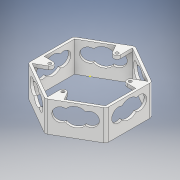
# Autodesk Inventor part: radar
Saved by Autodesk Inventor 2018 (Build 220112000, 112)
## iProperties
Created: 2017-05-12
Part Number: radar
Material: Default New Material(1)
Document SubType Name: Modeling
Designer: Vidal Villegas
Density: 1.13872 g/cm^3
Appearance: PLA
Mass: 28.1682 g
Surface Area: 205.405 cm^2
Volume: 24.7367 cm^3
Author: Vidal Villegas
Autodesk Inventor part; units mm, degrees
ref_plane "YZ Plane" through (0, 0, 0) normal (1, 0, 0) x (0, 1, 0)
ref_plane "XZ Plane" through (0, 0, 0) normal (0, 1, 0) x (-1, 0, 0)
ref_plane "XY Plane" through (0, 0, 0) normal (0, 0, 1) x (1, 0, 0)
sketch "Sketch1" plane through (0, 0, 0) normal (0, 0, 1) x (1, 0, 0)
  line L0 (-47.5136, -27.432) -> (-47.5136, 27.432)
  line L1 (-47.5136, 27.432) -> (0, 54.864)
  line L2 (0, 54.864) -> (47.5136, 27.432)
  line L3 (47.5136, 27.432) -> (47.5136, -27.432)
  line L4 (47.5136, -27.432) -> (0, -54.864)
  line L5 (0, -54.864) -> (-47.5136, -27.432)
  line L6 (0, 51.3999) -> (44.5136, 25.6999)
  line L7 (44.5136, 25.6999) -> (44.5136, -25.6999)
  line L8 (44.5136, -25.6999) -> (0, -51.3999)
  line L9 (0, -51.3999) -> (-44.5136, -25.6999)
  line L10 (-44.5136, -25.6999) -> (-44.5136, 25.6999)
  line L11 (-44.5136, 25.6999) -> (0, 51.3999)
  point P0 (0, 0)
  point P1 (0, 0)
  point P2 (0, 0)
  dimension "d0" = 54.864
  dimension "d1" = 3
  constraints: 24 end point, 2 coincident, 2 vertical alignment, 26 other
  measures "d0" distance of L0.start L0.end
  measures "d1" distance between parallel lines of L1 L11
extrude "Extrusion1" add sketch "Sketch1" along normal blind 37
sketch "Sketch2" plane through (0, 0, 37) normal (0, 0, 1) x (1, 0, 0)
  line L0 (0, 51.3999) -> (44.5136, 25.6999) projected
  line L1 (44.5136, 25.6999) -> (44.5136, -25.6999) projected
  line L2 (44.5136, -25.6999) -> (0, -51.3999) projected
  line L3 (0, -51.3999) -> (-44.5136, -25.6999) projected
  line L4 (-44.5136, -25.6999) -> (-44.5136, 25.6999) projected
  line L5 (-44.5136, 25.6999) -> (0, 51.3999) projected
  line L6 (-29.2636, 16.8954) -> (0, 33.7907)
  line L7 (0, 33.7907) -> (29.2636, 16.8954)
  line L8 (29.2636, 16.8954) -> (29.2636, -16.8954)
  line L9 (29.2636, -16.8954) -> (0, -33.7907)
  line L10 (0, -33.7907) -> (-29.2636, -16.8954)
  line L11 (-29.2636, -16.8954) -> (-29.2636, 16.8954)
  point P0 (0, 0)
  point P1 (0, 0)
  dimension "d4" = 15.25
  constraints: 12 end point, 1 coincident, 1 vertical alignment, 13 other
  measures "d4" distance between parallel lines of L8 L1
extrude "Extrusion2" add sketch "Sketch2" against normal blind 4
sketch "Sketch5" plane through (0, 0, 33) normal (0, 0, -1) x (-1, 0, 0)
  point P0 (0, 0)
sketch "Sketch6" plane through (0, 54.864, 37) normal (0.5, 0.8660254, 0) x (0.8660254, -0.5, 0)
  circle A0 centre (14.682, 14.5) radius 8.44
  circle A1 centre (40.182, 14.5) radius 8.44
  line L0 (0, 37) -> (54.864, 37) projected
  line L1 (0, 37) -> (0, 0) projected
  line L2 (54.864, 0) -> (0, 0) projected
  line L3 (54.864, 37) -> (54.864, 0) projected
  arc A2 (15.7427, 14.5) -> (39.1213, 14.5) centre (27.432, 15) ccw
  arc A3 (39.1213, 14.5) -> (15.7427, 14.5) centre (27.432, 14) ccw
  line L4 (27.432, 37) -> (27.432, 28.8885) construction
  point P0 (27.432, 37)
  dimension "d49" = 25.5
  dimension "d51" = 8.44
  dimension "d53" = 11.7
  dimension "d54" = 15
  dimension "d55" = 23
  dimension "d58" = 14.5
  constraints: 4 centre point, 4 point on circle, 2 end point, 2 equal radius, 2 vertical alignment, 1 horizontal alignment, 1 midpoint, 1 symmetric about line, 1 vertical
  measures "d49" distance of A0.centre A1.centre
  measures "d51" radius of A1
  measures "d53" radius of A2
  measures "d54" distance from line of A2.centre L2
  measures "d55" distance from line of L0 A3.centre
  measures "d58" distance from line of A0.centre L2
extrude "Extrusion3" cut sketch "Sketch6" against normal through all contours A0 A2 A3 | A0 A3 A1 A2 | A3 A2 A0 | A3 A2 A1 | A1 A2 A3
sketch "Sketch7" plane through (47.5136, -27.432, 0) normal (1, 0, 0) x (0, 0, -1)
  line L0 (0, 54.864) -> (0, 0) projected
  line L1 (0, 54.864) -> (-37, 54.864) projected
  line L2 (-37, 0) -> (-37, 54.864) projected
  line L3 (0, 0) -> (-37, 0) projected
  circle A0 centre (-22.5, 40.932) radius 8.5
  circle A1 centre (-22.5, 13.932) radius 8.5
  arc A2 (-17.5, 17.3946) -> (-17.5, 37.4694) centre (-13, 27.432) ccw
  arc A3 (-17.5, 37.4694) -> (-17.5, 17.3946) centre (-22, 27.432) ccw
  line L4 (0, 53.1319) -> (0, 1.7321) construction
  line L5 (0, 27.432) -> (3.1756, 27.432) construction
  point P0 (48.3121, 34.9149)
  point P1 (0, 27.432)
  dimension "d66" = 8.5
  dimension "d67" = 27
  dimension "d68" = 14.5
  dimension "d70" = 22
  dimension "d71" = 15
  dimension "d72" = 13
  constraints: 4 centre point, 4 point on circle, 2 end point, 2 equal radius, 2 horizontal alignment, 2 midpoint, 1 horizontal, 1 symmetric about line, 1 vertical alignment
  measures "d66" radius of A1
  measures "d67" distance of A0.centre A1.centre
  measures "d68" distance from line of L2 A0.centre
  measures "d70" diameter of A2
  measures "d71" distance from line of L2 A3.centre
  measures "d72" distance from line of A2.centre L0
extrude "Extrusion4" [suppressed]
sketch "Sketch8" plane through (47.5136, -27.432, 0) normal (0.5, -0.8660254, 0) x (0.8660254, 0.5, 0)
  line L0 (-54.864, 0) -> (0, 0) projected
  line L1 (-54.864, 0) -> (-54.864, 37) projected
  line L2 (0, 37) -> (-54.864, 37) projected
  line L3 (0, 0) -> (0, 37) projected
  line L4 (-54.864, 0) -> (0, 0) projected
  line L5 (-54.864, 0) -> (-54.864, 37) projected
  line L6 (0, 37) -> (-54.864, 37) projected
  line L7 (0, 0) -> (0, 37) projected
  circle A0 centre (13.932, 22.5) radius 8.5
  circle A1 centre (40.932, 22.5) radius 8.5
  line L8 (0, 37) -> (54.864, 37)
  line L9 (0, 37) -> (0, 0)
  line L10 (54.864, 0) -> (0, 0)
  line L11 (54.864, 37) -> (54.864, 0)
  arc A2 (17.3946, 17.5) -> (37.4694, 17.5) centre (27.432, 13) ccw
  arc A3 (37.4694, 17.5) -> (17.3946, 17.5) centre (27.432, 22) ccw
  line L12 (27.432, 37) -> (27.432, 28.8885) construction
  circle A4 centre (-13.932, 22.5) radius 8.5
  circle A5 centre (-40.932, 22.5) radius 8.5
  line L13 (0, 37) -> (-54.864, 37)
  line L14 (-54.864, 0) -> (0, 0)
  line L15 (-54.864, 37) -> (-54.864, 0)
  arc A6 (-37.4694, 17.5) -> (-17.3946, 17.5) centre (-27.432, 13) ccw
  arc A7 (-17.3946, 17.5) -> (-37.4694, 17.5) centre (-27.432, 22) ccw
  line L16 (-27.432, 37) -> (-27.432, 28.8885) construction
  line L17 (27.432, 0) -> (0, 0) projected
  line L18 (27.432, 0) -> (27.432, 37) projected
  line L19 (0, 37) -> (27.432, 37) projected
  line L20 (0, 0) -> (0, 37) projected
  line L21 (0, 0) -> (-54.864, 0) projected
  line L22 (-54.864, 37) -> (0, 37) projected
  line L23 (0, 0) -> (0, 37) projected
  point P0 (-27.432, 0)
  point P1 (27.432, 27)
  point P2 (-27.432, 27)
  dimension "d75" = 27
  dimension "d76" = 8.5
  dimension "d77" = 11
  dimension "d78" = 13
  dimension "d79" = 15
  dimension "d81" = 14.5
  dimension "d82" = 54.864
  dimension "d83" = 54.864
  constraints: 18 end point, 10 symmetric about line, 8 centre point, 8 point on circle, 2 collinear, 2 equal radius, 2 vertical, 2 vertical alignment, 1 horizontal, 1 horizontal alignment, 1 midpoint, 5 other
  measures "d75" distance of A0.centre A1.centre
  measures "d76" radius of A1
  measures "d77" radius of A2
  measures "d78" distance from line of A2.centre L10
  measures "d79" distance from line of L8 A3.centre
  measures "d81" distance from line of A0.centre L8
  measures "d82" distance between parallel lines of L9 L1
  measures "d83" distance between parallel lines of L3 L11
extrude "Extrusion5" [suppressed]
sketch "Sketch9" plane through (0, 0, 33) normal (0, 0, -1) x (-1, 0, 0)
  line L0 (0, 54.805) -> (-47.4625, 27.4025)
  line L1 (-47.4625, 27.4025) -> (-47.4625, -27.4025)
  line L2 (-47.4625, -27.4025) -> (0, -54.805)
  line L3 (-47.4625, 27.4025) -> (0, 54.805)
  line L4 (0, 54.805) -> (47.4625, 27.4025)
  line L5 (47.4625, 27.4025) -> (47.4625, -27.4025)
  line L6 (47.4625, -27.4025) -> (0, -54.805)
  line L7 (0, -54.805) -> (-47.4625, -27.4025)
  line L8 (-47.4625, -27.4025) -> (-47.4625, 27.4025)
  circle A0 centre (-29.8779, -21.75) radius 1.55
  circle A1 centre (-33.775, -15) radius 1.55
  circle A2 centre (-33.775, 15) radius 1.55
  circle A3 centre (-3.8971, -36.75) radius 1.55
  circle A4 centre (3.8971, -36.75) radius 1.55
  circle A5 centre (29.8779, -21.75) radius 1.55
  circle A6 centre (33.775, -15) radius 1.55
  circle A7 centre (33.775, 15) radius 1.55
  circle A8 centre (29.8779, 21.75) radius 1.55
  circle A9 centre (3.8971, 36.75) radius 1.55
  circle A10 centre (-3.8971, 36.75) radius 1.55
  line L9 (-33.775, 19.5) -> (0, 39) construction
  line L10 (0, 39) -> (33.775, 19.5) construction
  line L11 (33.775, 19.5) -> (33.775, -19.5) construction
  line L12 (33.775, -19.5) -> (0, -39) construction
  line L13 (0, -39) -> (-33.775, -19.5) construction
  line L14 (-33.775, -19.5) -> (-33.775, 19.5) construction
  circle A11 centre (-29.8779, 21.75) radius 1.55
  line L15 (-44.5136, -25.6999) -> (-44.5136, 25.6999) projected
  line L16 (-44.5136, 25.6999) -> (0, 51.3999) projected
  line L17 (0, 51.3999) -> (44.5136, 25.6999) projected
  line L18 (44.5136, 25.6999) -> (44.5136, -25.6999) projected
  line L19 (44.5136, -25.6999) -> (0, -51.3999) projected
  line L20 (0, -51.3999) -> (-44.5136, -25.6999) projected
  line L21 (47.5136, -27.432) -> (47.5136, 27.432) projected
  line L22 (47.5136, 27.432) -> (0, 54.864) projected
  line L23 (0, 54.864) -> (-47.5136, 27.432) projected
  line L24 (-47.5136, 27.432) -> (-47.5136, -27.432) projected
  line L25 (-47.5136, -27.432) -> (0, -54.864) projected
  line L26 (0, -54.864) -> (47.5136, -27.432) projected
  line L27 (44.5136, 25.6999) -> (44.5136, -25.6999) projected
  line L28 (44.5136, 11) -> (29.2636, 11)
  line L29 (29.2636, 11) -> (29.2636, -11)
  line L30 (29.2636, -11) -> (44.5136, -11)
  line L31 (44.5136, -11) -> (44.5136, 11)
  line L32 (44.5136, 0) -> (46.3422, 0) construction
  line L33 (0, -33.7907) -> (-29.2636, -16.8954) construction
  line L34 (-29.2636, -16.8954) -> (-29.2636, 16.8954) construction
  line L35 (-29.2636, 16.8954) -> (-18.084, 23.3499) construction
  line L36 (0, 33.7907) -> (29.2636, 16.8954) construction
  line L37 (29.2636, 16.8954) -> (29.2636, -16.8954) construction
  line L38 (29.2636, -16.8954) -> (18.084, -23.3499) construction
  line L39 (0, -51.3999) -> (-44.5136, -25.6999) construction
  line L40 (18.8046, -40.543) -> (0, -51.3999) construction
  line L41 (44.5136, -25.6999) -> (25.709, -36.5568) construction
  line L42 (44.5136, 25.6999) -> (44.5136, -25.6999) construction
  line L43 (0, 51.3999) -> (44.5136, 25.6999) construction
  line L44 (-18.8046, 40.543) -> (0, 51.3999) construction
  line L45 (-44.5136, 25.6999) -> (-25.709, 36.5568) construction
  line L46 (-44.5136, -25.6999) -> (-44.5136, 25.6999) construction
  line L47 (12.7305, 44.0499) -> (5.1055, 30.843)
  line L48 (29.2636, 16.8954) -> (0, 33.7907) projected
  line L49 (24.1581, 19.843) -> (31.7831, 33.0499)
  line L50 (31.7831, 33.0499) -> (12.7305, 44.0499)
  line L51 (5.1055, 30.843) -> (24.1581, 19.843)
  line L52 (22.2568, 38.5499) -> (22.6365, 39.2076)
  line L53 (0, 51.3999) -> (44.5136, 25.6999) projected
  line L54 (0, 33.7907) -> (29.2636, 16.8954) projected
  line L55 (0, 0) -> (0, -5.712) construction
  line L56 (0, 0) -> (4.8403, -2.7945) construction
  line L57 (29.2636, 16.8954) -> (29.2636, -16.8954) construction
  line L58 (-44.5136, 11) -> (-29.2636, 11)
  line L59 (-29.2636, 11) -> (-29.2636, -11)
  line L60 (-29.2636, -11) -> (-44.5136, -11)
  line L61 (-44.5136, -11) -> (-44.5136, 11)
  line L62 (-31.7831, -33.0499) -> (-24.1581, -19.843)
  line L63 (-5.1055, -30.843) -> (-12.7305, -44.0499)
  line L64 (-12.7305, -44.0499) -> (-31.7831, -33.0499)
  line L65 (-24.1581, -19.843) -> (-5.1055, -30.843)
  line L66 (-22.2568, -38.5499) -> (-22.6365, -39.2076)
  line L67 (0, -54.864) -> (47.5136, -27.432) construction
  line L68 (23.7568, -41.148) -> (25.1641, -43.5855) construction
  line L69 (29.2636, -16.8954) -> (0, -33.7907) projected
  line L70 (24.1581, -19.843) -> (31.7831, -33.0499)
  line L71 (25.709, -36.5568) -> (0, -51.3999) projected
  line L72 (12.7305, -44.0499) -> (5.1055, -30.843)
  line L73 (24.1581, -19.843) -> (5.1055, -30.843)
  line L74 (12.7305, -44.0499) -> (31.7831, -33.0499)
  line L75 (44.5136, -25.6999) -> (0, -51.3999) projected
  line L76 (0, 0) -> (6.6102, 3.8164) construction
  line L77 (0, 51.3999) -> (-44.5136, 25.6999)
  line L78 (0, 33.7907) -> (-29.2636, 16.8954) construction
  line L79 (-5.1055, 30.843) -> (-12.7305, 44.0499)
  line L80 (-31.7831, 33.0499) -> (-24.1581, 19.843)
  line L81 (-5.1055, 30.843) -> (-24.1581, 19.843)
  line L82 (-5.1055, 30.843) -> (-24.1581, 19.843)
  line L83 (-29.2636, 16.8954) -> (0, 33.7907) projected
  line L84 (-24.1581, 19.843) -> (-31.7831, 33.0499)
  line L85 (-24.1581, 19.843) -> (-31.7831, 33.0499)
  line L86 (-31.7831, 33.0499) -> (-12.7305, 44.0499)
  line L87 (-12.7305, 44.0499) -> (-5.1055, 30.843)
  line L88 (5.1055, -30.843) -> (24.1581, -19.843)
  line L89 (0, -33.7907) -> (29.2636, -16.8954) projected
  line L90 (31.7831, -33.0499) -> (24.1581, -19.843)
  line L91 (31.7831, -33.0499) -> (12.7305, -44.0499)
  line L92 (12.7305, -44.0499) -> (5.1055, -30.843)
  line L93 (5.1055, 30.843) -> (24.1581, 19.843)
  line L94 (24.1581, 19.843) -> (31.7831, 33.0499)
  line L95 (41.3094, 27.5499) -> (29.4425, 34.4013) projected
  line L96 (31.7831, 33.0499) -> (12.7305, 44.0499)
  line L97 (12.7305, 44.0499) -> (5.1055, 30.843)
  line L98 (-5.1055, 30.843) -> (-12.7305, 44.0499)
  line L99 (-12.7305, 44.0499) -> (-31.7831, 33.0499)
  line L100 (-31.7831, 33.0499) -> (-24.1581, 19.843)
  line L101 (-24.1581, 19.843) -> (-5.1055, 30.843)
  line L102 (-5.1055, -30.843) -> (-24.1581, -19.843)
  line L103 (-24.1581, -19.843) -> (-31.7831, -33.0499)
  line L104 (0, -33.7907) -> (-29.2636, -16.8954) projected
  line L105 (-31.7831, -33.0499) -> (-12.7305, -44.0499)
  line L106 (-12.7305, -44.0499) -> (-5.1055, -30.843)
  line L107 (18.8046, -40.543) -> (11.1796, -27.3361) projected
  line L108 (11.1796, -27.3361) -> (0, -33.7907) projected
  line L109 (-18.084, 23.3499) -> (-25.709, 36.5568) projected
  line L110 (18.084, -23.3499) -> (25.709, -36.5568) projected
  line L111 (-18.8046, 40.543) -> (-11.1796, 27.3361) projected
  line L112 (-11.1796, 27.3361) -> (0, 33.7907) projected
  point P0 (-44.5136, 0)
  point P1 (-44.5136, 0)
  dimension "d86" = 3.1
  dimension "d87" = 39
  dimension "d88" = 4.5
  dimension "d89" = 4.5
  dimension "d90" = 4.5
  dimension "d91" = 4.5
  dimension "d92" = 4.5
  dimension "d93" = 4.5
  dimension "d94" = 4.5
  dimension "d95" = 4.5
  dimension "d96" = 4.5
  dimension "d97" = 4.5
  dimension "d98" = 4.5
  dimension "d99" = 4.5
  dimension "d100" = 22
  dimension "d101" = 22
  dimension "d102" = 22
  constraints: 136 end point, 22 perpendicular, 22 point on line, 16 symmetric about line, 12 centre point, 11 equal radius, 9 collinear, 5 parallel, 3 vertical, 2 coincident, 2 horizontal, 1 midpoint, 29 other
  measures "d86" diameter of A0
  measures "d87" distance of L13.end L9.start
  measures "d88" distance of A1.centre L13.end
  measures "d89" distance of A0.centre L13.end
  measures "d90" distance of L9.start A2.centre
  measures "d91" distance of A3.centre L12.end
  measures "d92" distance of L12.end A4.centre
  measures "d93" distance of L11.end A5.centre
  measures "d94" distance of L9.end A10.centre
  measures "d95" distance of A9.centre L9.end
  measures "d96" distance of L10.end A8.centre
  measures "d97" distance of L9.start A11.centre
  measures "d98" distance of L10.end A7.centre
  measures "d99" distance of A6.centre L11.end
  measures "d100" distance between parallel lines of L28 L30
  measures "d101" distance between parallel lines of L47 L49
  measures "d102" distance between parallel lines of L70 L72
hole "Hole3" at (-33.775, 15, 33) at (-29.8779, 21.75, 33) at (-33.775, -15, 33) at (-29.8779, -21.75, 33) at (-3.8971, -36.75, 33) at (3.8971, -36.75, 33) at (29.8779, -21.75, 33) at (33.775, -15, 33) at (33.775, 15, 33) at (29.8779, 21.75, 33) at (3.8971, 36.75, 33) at (-3.8971, 36.75, 33) direction (0, 0, 1) diameter 3.7 end through all
extrude "Extrusion6" cut sketch "Sketch9" against normal through all contours L30 L29 L28 L18
extrude "Extrusion7" cut sketch "Sketch9" against normal through all contours L15 L58 L59 L60
extrude "Extrusion8" cut sketch "Sketch9" against normal through all contours L17 L49 L48 L47
extrude "Extrusion9" cut sketch "Sketch9" against normal through all contours L72 L69 L107 L19 | L107 L69 L110 L19 | L110 L69 L70 L19
extrude "Extrusion10" cut sketch "Sketch9" against normal through all contours L16 L109 L81 L80 | L16 L111 L81 L109 | L16 L79 L81 L111
extrude "Extrusion11" cut sketch "Sketch9" against normal through all contours L62 L65 L63 L20
pattern_circular "Circular Pattern1" count 6 over 360 about axis through (0, 0, -10) along (0, 0, 1) of "Extrusion3"
sketch "Sketch10" plane through (0, 0, 33) normal (0, 0, -1) x (-1, 0, 0)
  line L0 (24.1581, -19.843) -> (31.7831, -33.0499) projected
  line L1 (44.5136, -25.6999) -> (31.7831, -33.0499) projected
  line L2 (44.5136, -11) -> (44.5136, -25.6999) projected
  line L3 (44.5136, -11) -> (29.2636, -11) projected
  line L4 (29.2636, -11) -> (29.2636, -16.8954) projected
  line L5 (29.2636, -16.8954) -> (24.1581, -19.843) projected
  circle A0 centre (33.775, -15) radius 1.85 projected
  circle A1 centre (29.8779, -21.75) radius 1.85 projected
  line L6 (-5.1055, -30.843) -> (-12.7305, -44.0499) projected
  line L7 (0, -51.3999) -> (-12.7305, -44.0499) projected
  line L8 (12.7305, -44.0499) -> (0, -51.3999) projected
  line L9 (12.7305, -44.0499) -> (5.1055, -30.843) projected
  line L10 (5.1055, -30.843) -> (0, -33.7907) projected
  line L11 (0, -33.7907) -> (-5.1055, -30.843) projected
  circle A2 centre (-3.8971, -36.75) radius 1.85 projected
  circle A3 centre (3.8971, -36.75) radius 1.85 projected
  circle A4 centre (-33.775, -15) radius 1.85 projected
  circle A5 centre (-29.8779, -21.75) radius 1.85 projected
  line L12 (-31.7831, -33.0499) -> (-24.1581, -19.843) projected
  line L13 (-24.1581, -19.843) -> (-29.2636, -16.8954) projected
  line L14 (-29.2636, -16.8954) -> (-29.2636, -11) projected
  line L15 (-29.2636, -11) -> (-44.5136, -11) projected
  line L16 (-44.5136, -25.6999) -> (-44.5136, -11) projected
  line L17 (-31.7831, -33.0499) -> (-44.5136, -25.6999) projected
  line L18 (-24.1581, 19.843) -> (-31.7831, 33.0499) projected
  line L19 (-44.5136, 25.6999) -> (-31.7831, 33.0499) projected
  line L20 (-44.5136, 11) -> (-44.5136, 25.6999) projected
  line L21 (-44.5136, 11) -> (-29.2636, 11) projected
  line L22 (-29.2636, 11) -> (-29.2636, 16.8954) projected
  line L23 (-29.2636, 16.8954) -> (-24.1581, 19.843) projected
  circle A6 centre (-33.775, 15) radius 1.85 projected
  circle A7 centre (-29.8779, 21.75) radius 1.85 projected
  circle A8 centre (3.8971, 36.75) radius 1.85 projected
  circle A9 centre (-3.8971, 36.75) radius 1.85 projected
  line L24 (-12.7305, 44.0499) -> (-5.1055, 30.843) projected
  line L25 (-5.1055, 30.843) -> (0, 33.7907) projected
  line L26 (0, 33.7907) -> (5.1055, 30.843) projected
  line L27 (5.1055, 30.843) -> (12.7305, 44.0499) projected
  line L28 (0, 51.3999) -> (12.7305, 44.0499) projected
  line L29 (-12.7305, 44.0499) -> (0, 51.3999) projected
  line L30 (31.7831, 33.0499) -> (24.1581, 19.843) projected
  line L31 (24.1581, 19.843) -> (29.2636, 16.8954) projected
  line L32 (29.2636, 16.8954) -> (29.2636, 11) projected
  line L33 (29.2636, 11) -> (44.5136, 11) projected
  line L34 (44.5136, 25.6999) -> (44.5136, 11) projected
  line L35 (31.7831, 33.0499) -> (44.5136, 25.6999) projected
  circle A10 centre (33.775, 15) radius 1.85 projected
  circle A11 centre (29.8779, 21.75) radius 1.85 projected
  line L36 (29.2636, -11) -> (29.2636, -16.8954) projected
  line L37 (29.2636, -16.8954) -> (44.5136, -25.6999)
  line L38 (0, -33.7907) -> (0, -51.3999)
  line L39 (-29.2636, -16.8954) -> (-44.5136, -25.6999)
  line L40 (-29.2636, 16.8954) -> (-29.2636, 11) projected
  line L41 (-29.2636, 16.8954) -> (-44.5136, 25.6999)
  line L42 (5.1055, 30.843) -> (0, 33.7907) projected
  line L43 (0, 33.7907) -> (0, 51.3999)
  line L44 (29.2636, 16.8954) -> (44.5136, 25.6999)
  point P0 (0, 0)
  constraints: 12 end point, 1 collinear, 1 parallel, 1 point on line
extrude "Extrusion12" cut sketch "Sketch10" against normal blind 10 contours L5 L37 L1 L0 | L10 L9 L8 L38 | L17 L39 L13 L12 | L16 L15 L14 L39 | L23 L41 L19 L18 | L35 L44 L31 L30 | L34 L33 L32 L44
sketch "Sketch11" plane through (0, 0, 33) normal (0, 0, -1) x (-1, 0, 0)
  circle A0 centre (3.8971, 36.75) radius 1.85 projected
  circle A1 centre (-3.8971, 36.75) radius 1.85 projected
  line L0 (-12.7305, 44.0499) -> (-5.1055, 30.843) projected
  line L1 (-5.1055, 30.843) -> (0, 33.7907) projected
  line L2 (0, 33.7907) -> (5.1055, 30.843) projected
  line L3 (5.1055, 30.843) -> (12.7305, 44.0499) projected
  line L4 (0, 51.3999) -> (12.7305, 44.0499) projected
  line L5 (-12.7305, 44.0499) -> (0, 51.3999) projected
  line L6 (0, 33.7907) -> (0, 51.3999)
  point P0 (0, 0)
  constraints: 2 end point, 1 vertical
extrude "Extrusion13" cut sketch "Sketch11" against normal through all contours L5 L6 L1 L0
fillet "Fillet1" radius 4 6 edges at (47.5136, 27.432, 18.5) (47.5136, -27.432, 18.5) (0, -54.864, 18.5) (-47.5136, -27.432, 18.5) (-47.5136, 27.432, 18.5) (0, 54.864, 18.5)
fillet "Fillet2" radius 4 8 edges at (29.2636, 11, 35) (29.2636, 16.8954, 35) (-5.1055, 30.843, 35) (0, 33.7907, 35) (-29.2636, -16.8954, 35) (-29.2636, -11, 35) (0, -33.7907, 35) (5.1055, -30.843, 35)
sketch "Sketch14" plane through (-47.5136, -25.1226, 0) normal (-1, 0, 0) x (0, 0, 1)
  arc A0 (15.1224, 16.472) -> (29.8776, 16.472) centre (22.5, 12.3726) ccw projected
  arc A1 (15.1224, 33.7732) -> (15.1224, 16.472) centre (23, 25.1226) ccw projected
  arc A2 (29.8776, 33.7732) -> (15.1224, 33.7732) centre (22.5, 37.8726) ccw projected
  arc A3 (29.8776, 16.472) -> (29.8776, 33.7732) centre (22, 25.1226) ccw projected
  point P0 (0, 25.1226)
sketch "Sketch12" plane through (2, 53.7093, 37) normal (0.5, 0.8660254, 0) x (0.8660254, -0.5, 0)
  arc A0 (33.7732, 21.8776) -> (16.472, 21.8776) centre (25.1226, 14) ccw projected
  arc A1 (16.472, 21.8776) -> (16.472, 7.1224) centre (12.3726, 14.5) ccw projected
  arc A2 (16.472, 7.1224) -> (33.7732, 7.1224) centre (25.1226, 15) ccw projected
  arc A3 (33.7732, 7.1224) -> (33.7732, 21.8776) centre (37.8726, 14.5) ccw projected
  point P0 (25.1226, 37)
sketch "Sketch13" plane through (-2, 53.7093, 37) normal (-0.5, 0.8660254, 0) x (0.8660254, 0.5, 0)
  arc A0 (-16.472, 7.1224) -> (-16.472, 21.8776) centre (-12.3726, 14.5) ccw projected
  arc A1 (-33.7732, 7.1224) -> (-16.472, 7.1224) centre (-25.1226, 15) ccw projected
  arc A2 (-33.7732, 21.8776) -> (-33.7732, 7.1224) centre (-37.8726, 14.5) ccw projected
  arc A3 (-16.472, 21.8776) -> (-33.7732, 21.8776) centre (-25.1226, 14) ccw projected
  point P0 (-25.1226, 37)
sketch "Sketch15" plane through (-45.5136, -28.5867, 0) normal (-0.5, -0.8660254, 0) x (0.8660254, -0.5, 0)
  arc A0 (33.7732, 15.1224) -> (33.7732, 29.8776) centre (37.8726, 22.5) ccw projected
  arc A1 (16.472, 15.1224) -> (33.7732, 15.1224) centre (25.1226, 23) ccw projected
  arc A2 (16.472, 29.8776) -> (16.472, 15.1224) centre (12.3726, 22.5) ccw projected
  arc A3 (33.7732, 29.8776) -> (16.472, 29.8776) centre (25.1226, 22) ccw projected
  point P0 (25.1226, 0)
sketch "Sketch17" plane through (47.5136, -25.1226, 0) normal (1, 0, 0) x (0, 0, -1)
  arc A0 (-15.1224, 33.7732) -> (-29.8776, 33.7732) centre (-22.5, 37.8726) ccw projected
  arc A1 (-15.1224, 16.472) -> (-15.1224, 33.7732) centre (-23, 25.1226) ccw projected
  arc A2 (-29.8776, 16.472) -> (-15.1224, 16.472) centre (-22.5, 12.3726) ccw projected
  arc A3 (-29.8776, 33.7732) -> (-29.8776, 16.472) centre (-22, 25.1226) ccw projected
  point P0 (0, 25.1226)
sketch "Sketch16" plane through (2, -53.7093, 0) normal (0.5, -0.8660254, 0) x (0.8660254, 0.5, 0)
  arc A0 (33.7732, 15.1224) -> (33.7732, 29.8776) centre (37.8726, 22.5) ccw projected
  arc A1 (16.472, 15.1224) -> (33.7732, 15.1224) centre (25.1226, 23) ccw projected
  arc A2 (16.472, 29.8776) -> (16.472, 15.1224) centre (12.3726, 22.5) ccw projected
  arc A3 (33.7732, 29.8776) -> (16.472, 29.8776) centre (25.1226, 22) ccw projected
  point P0 (25.1226, 0)
equation "\"d83\" = d82"
equation "\"d89\" = d88"
equation "\"d90\" = d88"
equation "\"d91\" = d89"
equation "\"d92\" = d88"
equation "\"d93\" = d88"
equation "\"d94\" = d88"
equation "\"d95\" = d88"
equation "\"d96\" = d88"
equation "\"d97\" = d90"
equation "\"d98\" = d96"
equation "\"d99\" = d93"
equation "\"d101\" = d100"
equation "\"d102\" = d100"
body "Solid1"
